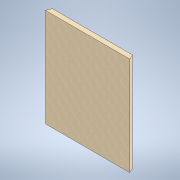
# Autodesk Inventor part: PlatteAussenZweiSeiten
Saved by Autodesk Inventor 2020.3 (Build 243373010, 373A)
## iProperties
Created: 2021-02-12
Part Number: PlatteAussenZweiSeiten
Material: Generisch
Document SubType Name: Modeling
Designer: Stefan
Density: 1 g/cm^3
Appearance: Pappel
Author: Stefan
Autodesk Inventor part; units mm, degrees
ref_plane "YZ Plane" through (0, 0, 0) normal (1, 0, 0) x (0, 1, 0)
ref_plane "XZ Plane" through (0, 0, 0) normal (0, 1, 0) x (-1, 0, 0)
ref_plane "XY Plane" through (0, 0, 0) normal (0, 0, 1) x (1, 0, 0)
sketch "Skizze1" plane through (0, 0, 0) normal (0, 0, 1) x (1, 0, 0)
  line L0 (-149.1768, 16.7418) -> (13.9312, 16.7418)
  line L1 (13.9312, 16.7418) -> (13.9312, -183.2582)
  line L2 (13.9312, -183.2582) -> (-149.1768, -183.2582)
  line L3 (-149.1768, -183.2582) -> (-149.1768, 16.7418)
  point P0 (0, 0)
  point P1 (13.9312, 16.7418)
  dimension "d0" = 163.108
  dimension "d1" = 200
  dimension "d2" = 13.9312
  dimension "d3" = 16.7418
  dimension "d4" = 0
  dimension "d5" = 0
  dimension "d6" = 0
  dimension "d7" = 200
  dimension "d8" = 163.108
  dimension "d9" = 0
  dimension "d10" = 163.108
  dimension "d11" = 200
  constraints: 8 end point, 2 parallel, 1 horizontal, 1 vertical
  measures "d0" distance between parallel lines of L1 L3
  measures "d1" distance between parallel lines of L0 L2
  measures "d2" distance from line of point (0, 0) L1
  measures "d3" distance from line of point (0, 0) L0
  measures "d4" distance from line of L0.end L1
  measures "d5" distance from line of L1.start L0
  measures "d6" distance from line of L2.start L1
  measures "d7" distance from line of L1.end L0
  measures "d8" distance from line of L0.start L1
  measures "d9" distance from line of L3.end L0
  measures "d10" distance from line of L2.end L1
  measures "d11" distance from line of L3.start L0
extrude "Extrusion1" add sketch "Skizze1" along normal blind 10
sketch "Skizze2" plane through (-149.1768, -183.2582, 0) normal (0, -1, 0) x (1, 0, 0)
  line L0 (0, 10) -> (163.108, 10) projected
  line L1 (0, 0) -> (0, 10)
  line L2 (0, 10) -> (-4.1421, 10)
  line L3 (0, 0) -> (-4.1421, 10)
  line L4 (163.108, 0) -> (163.108, 10) projected
  line L5 (163.108, 0) -> (163.108, 10)
  line L6 (163.108, 10) -> (167.2501, 10)
  line L7 (163.108, 0) -> (167.2501, 10)
  point P0 (149.1768, 0)
  dimension "d14" = 22.5
  dimension "d15" = 22.5
  constraints: 12 end point, 2 perpendicular, 1 collinear, 1 vertical
  measures "d14" angle of L1 L3
  measures "d15" angle of L4 L7
extrude "Extrusion2" add sketch "Skizze2" against normal up to surface (200 mm away)
